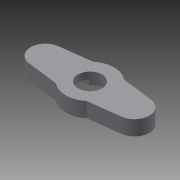
# Autodesk Inventor part: ServoHornPocket
Saved by Autodesk Inventor 2014 SP1 (Build 180222100, 222)
## iProperties
Created: 2017-01-17
Part Number: ServoHornPocket
Material: Generic
Document SubType Name: Modeling
Designer: danielsikar
Density: 1 g/cm^3
Appearance: Default
Author: danielsikar
Autodesk Inventor part; units mm, degrees
ref_plane "YZ Plane" through (0, 0, 0) normal (1, 0, 0) x (0, 1, 0)
ref_plane "XZ Plane" through (0, 0, 0) normal (0, 1, 0) x (-1, 0, 0)
ref_plane "XY Plane" through (0, 0, 0) normal (0, 0, 1) x (1, 0, 0)
sketch "bASE" plane through (0, 0, 0) normal (0, 0, 1) x (1, 0, 0)
  arc A0 (-16.7865, 2.679) -> (-16.7865, -2.679) centre (-16.45, 0) ccw
  arc A1 (16.7865, -2.679) -> (16.7865, 2.679) centre (16.45, 0) ccw
  line L0 (4.4678, -4.2262) -> (16.7865, -2.679)
  line L1 (4.4678, 4.2262) -> (16.7865, 2.679)
  line L2 (-4.4678, 4.2262) -> (-16.7865, 2.679)
  line L3 (-4.4678, -4.2262) -> (-16.7865, -2.679)
  arc A2 (-4.4678, -4.2262) -> (4.4678, -4.2262) centre (0, 0) ccw
  arc A3 (4.4678, 4.2262) -> (-4.4678, 4.2262) centre (0, 0) ccw
  point P0 (0, 4.2262)
  dimension "d20" = 5.4
  dimension "d21" = 5.4
  constraints: 8 end point, 8 point on circle, 4 centre point, 4 tangent, 1 coincident, 1 vertical alignment
  measures "d20" diameter of A0
  measures "d21" diameter of A1
sketch "Coupling" plane through (0, 0, 0) normal (0, 0, 1) x (1, 0, 0)
  line L0 (-4.4678, 4.2262) -> (-16.7865, 2.679) projected
  arc A0 (4.4678, 4.2262) -> (-4.4678, 4.2262) centre (0, 0) ccw projected
  line L1 (4.4678, 4.2262) -> (16.7865, 2.679) projected
  arc A1 (16.7865, -2.679) -> (16.7865, 2.679) centre (16.45, 0) ccw projected
  line L2 (4.4678, -4.2262) -> (16.7865, -2.679) projected
  arc A2 (-4.4678, -4.2262) -> (4.4678, -4.2262) centre (0, 0) ccw projected
  line L3 (-4.4678, -4.2262) -> (-16.7865, -2.679) projected
  arc A3 (-16.7865, 2.679) -> (-16.7865, -2.679) centre (-16.45, 0) ccw projected
  line L4 (17.1339, 5.4452) -> (5.7046, 6.8807)
  arc A4 (5.7046, 6.8807) -> (-5.7046, 6.8807) centre (0, 0) ccw
  line L5 (-5.7046, 6.8807) -> (-17.1339, 5.4452)
  arc A5 (-17.1339, 5.4452) -> (-17.1339, -5.4452) centre (-16.45, 0) ccw
  line L6 (-17.1339, -5.4452) -> (-5.7046, -6.8807)
  arc A6 (-5.7046, -6.8807) -> (5.7046, -6.8807) centre (0, 0) ccw
  line L7 (5.7046, -6.8807) -> (17.1339, -5.4452)
  arc A7 (17.1339, -5.4452) -> (17.1339, 5.4452) centre (16.45, 0) ccw
  constraints: 8 end point, 8 point on circle, 4 centre point, 7 other
extrude "Extrusion7" add sketch "Coupling" along normal blind 5.5 contours A0 L1 A1 L2 A2 L3 A3 L0 | A7 L7 A6 L6 A5 L5 A4 L4
extrude "Extrusion8" cut sketch "bASE" along normal blind 3
sketch "Sketch8" plane through (0, 0, 3) normal (0, 0, -1) x (-1, 0, 0)
  arc A0 (-4.4678, -4.2262) -> (4.4678, -4.2262) centre (0, 0) ccw projected
  circle A1 centre (0, 0) radius 4.45
  dimension "d26" = 8.9
  constraints: 1 centre point, 1 coincident
  measures "d26" diameter of A1
extrude "Extrusion9" cut sketch "Sketch8" against normal blind 3
body "Solid3"
